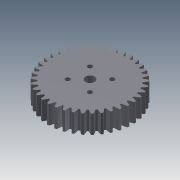
# Autodesk Inventor part: Spur Gear2
Saved by Autodesk Inventor 2015 (Build 190159000, 159)
## iProperties
Created: 2014-08-31
Part Number: Spur Gear2
Material: Steel
Document SubType Name: Modeling
Designer: shohei
Categories: <?xml version="1.0" encoding="UTF-16"?> <MemberInstance><Categories><FamilyTemplate><FamilyTemplateParameter ValueType="xs:double" Id="1" ObjectReferenceKey="da_z" ObjectType="kUserParameterObject"/><FamilyTemplateParameter ValueType="xs:double" Id="2" ObjectReferenceKey="da_b" ObjectType="kUserParameterObject"/><FamilyTemplateParameter ValueType="xs:double" Id="3" ObjectReferenceKey="da_beta" ObjectType="kUserParameterObject"/><FamilyTemplateParameter ValueType="xs:double" Id="4" ObjectReferenceKey="da_da" ObjectType="kUserParameterObject"/><FamilyTemplateParameter ValueType="xs:double" Id="5" ObjectReferenceKey="da_aw" ObjectType="kUserParameterObject"/><FamilyTemplateParameter ValueType="xs:string" Id="6" ObjectReferenceKey="EAIAABAAAACIAQAAAAAAAIAAAAAAAAAA" ObjectType="83910656" SubObjectId="SurfaceGeometry"/></FamilyTemplate><ParamToTemplateMap><ParamToTemplate CategoryParameter="//CategoryParameter[@InternalName='046C89C9-8512-4d59-83FE-43B91F4F132A']" TemplateParameter="1"/><ParamToTemplate CategoryParameter="//CategoryParameter[@InternalName='2552DF32-E462-4b46-AEBF-C6C7768E72AC']" TemplateParameter="2"/><ParamToTemplate CategoryParameter="//CategoryParameter[@InternalName='C9EE641D-15FC-4fae-A226-E94C4372FDD7']" TemplateParameter="3"/><ParamToTemplate><ParamToTemplate CategoryParameter="//CategoryParameter[@InternalName='00B6519A-459B-49c7-AD84-2E56D39A5744']" ConstantValue="0.112596"/></ParamToTemplate><ParamToTemplate><ParamToTemplate CategoryParameter="//CategoryParameter[@InternalName='04B31F0E-C7A6-4894-AA32-9629BEFACF47']" ConstantValue="1.000000"/></ParamToTemplate><ParamToTemplate><ParamToTemplate CategoryParameter="//CategoryParameter[@InternalName='43CBEC2E-7847-49e7-A936-2F7889FCB2D9']" ConstantValue="0.250000"/></ParamToTemplate><ParamToTemplate><ParamToTemplate CategoryParameter="//CategoryParameter[@InternalName='B1EFC894-105D-4ebd-86BF-FA20ED196853']" ConstantValue="0.350000"/></ParamToTemplate><ParamToTemplate><ParamToTemplate CategoryParameter="//CategoryParameter[@InternalName='51175063-3D10-4879-93E8-6246FE8B403D']" ConstantValue="2060000000.000000"/></ParamToTemplate><ParamToTemplate><ParamToTemplate CategoryParameter="//CategoryParameter[@InternalName='A3A52E27-4454-46a9-B0BD-C932399B70AF']" ConstantValue="0.300000"/></ParamToTemplate><ParamToTemplate><ParamToTemplate CategoryParameter="//CategoryParameter[@InternalName='91B76062-C214-41d9-B1B9-14D2AB99603D']" ConstantValue="0.225000"/></ParamToTemplate><ParamToTemplate><ParamToTemplate CategoryParameter="//CategoryParameter[@InternalName='374E806E-8B8A-4dda-A9AA-1039D6500AD2']" ConstantValue="4.444444"/></ParamToTemplate><ParamToTemplate><ParamToTemplate CategoryParameter="//CategoryParameter[@InternalName='2D373A89-B862-43d6-8D0B-0CBF12AB9F6C']" ConstantValue="0.349066"/></ParamToTemplate><ParamToTemplate CategoryParameter="//CategoryParameter[@InternalName='37777632-D6A2-4fac-9D53-DB8ACD95C989']" TemplateParameter="4"/><ParamToTemplate CategoryParameter="//CategoryParameter[@InternalName='FD1017F1-B727-4f7e-9707-0F86F1FF9423']" TemplateParameter="5"/><ParamToTemplate><ParamToTemplate CategoryParameter="//CategoryParameter[@InternalName='9E1B4470-B2D3-4ff1-B813-535BB4CDF51A']" ConstantValue="3520000.000000"/></ParamToTemplate><ParamToTemplate><ParamToTemplate CategoryParameter="//CategoryParameter[@InternalName='F8452263-BFF6-458c-9FB1-07C4B99E95CD']" ConstantValue="11400000.000000"/></ParamToTemplate><ParamToTemplate><ParamToTemplate CategoryParameter="//CategoryParameter[@InternalName='3E3BB259-FD49-497f-8171-6EBC954A3479']" ConstantValue="2.000000"/></ParamToTemplate><ParamToTemplate CategoryParameter="//CategoryParameter[@InternalName='27C3BAF2-7550-4e4b-AE2C-0DB134B7D9B7']" TemplateParameter="6"/></ParamToTemplateMap><Category DisplayName="Gear" InternalName="DC85795E-93AB-48d5-8EEE-5A27447B64BD" Mnemonic="Gear"><CategoryParameter DisplayName="z" InternalName="046C89C9-8512-4d59-83FE-43B91F4F132A" Mnemonic="z"/><CategoryParameter DisplayName="b" InternalName="2552DF32-E462-4b46-AEBF-C6C7768E72AC" Mnemonic="b"/><CategoryParameter DisplayName="||b|" InternalName="C9EE641D-15FC-4fae-A226-E94C4372FDD7" Mnemonic="beta"/><CategoryParameter DisplayName="x" InternalName="00B6519A-459B-49c7-AD84-2E56D39A5744" Mnemonic="x"/><CategoryParameter DisplayName="a*" InternalName="04B31F0E-C7A6-4894-AA32-9629BEFACF47" Mnemonic="a"/><CategoryParameter DisplayName="c*" InternalName="43CBEC2E-7847-49e7-A936-2F7889FCB2D9" Mnemonic="c"/><CategoryParameter DisplayName="r|.f|*" InternalName="B1EFC894-105D-4ebd-86BF-FA20ED196853" Mnemonic="rf"/><CategoryParameter DisplayName="E" InternalName="51175063-3D10-4879-93E8-6246FE8B403D" Mnemonic="E"/><CategoryParameter DisplayName="||m|" InternalName="A3A52E27-4454-46a9-B0BD-C932399B70AF" Mnemonic="mi"/><Category DisplayName="SpurGear" InternalName="26C5A22E-A91E-4dfd-A3B3-23CCAFAE1764" Mnemonic="SpurGear"><CategoryParameter DisplayName="m" InternalName="91B76062-C214-41d9-B1B9-14D2AB99603D" Mnemonic="m"/><CategoryParameter DisplayName="P" InternalName="374E806E-8B8A-4dda-A9AA-1039D6500AD2" Mnemonic="PP"/><CategoryParameter DisplayName="||a|" InternalName="2D373A89-B862-43d6-8D0B-0CBF12AB9F6C" Mnemonic="alpha"/><CategoryParameter DisplayName="d|.a|" InternalName="37777632-D6A2-4fac-9D53-DB8ACD95C989" Mnemonic="da"/><CategoryParameter DisplayName="a|.w|" InternalName="FD1017F1-B727-4f7e-9707-0F86F1FF9423" Mnemonic="aw"/><CategoryParameter DisplayName="||s||.Flim|" InternalName="9E1B4470-B2D3-4ff1-B813-535BB4CDF51A" Mnemonic="sFlim"/><CategoryParameter DisplayName="||s||.Hlim|" InternalName="F8452263-BFF6-458c-9FB1-07C4B99E95CD" Mnemonic="sHlim"/><CategoryParameter DisplayName="type" InternalName="3E3BB259-FD49-497f-8171-6EBC954A3479" Mnemonic="type"/><CategoryParameter DisplayName="PitchDiameter" InternalName="27C3BAF2-7550-4e4b-AE2C-0DB134B7D9B7" Mnemonic="IDS_PITCHDIAM"/></Category></Category></Categories></MemberInstance>
Density: 1 g/cm^3
Appearance: Steel
CustomPartVersion: 1
Author: shohei
Autodesk Inventor part; units mm, degrees
(part 1 of 2)
ref_plane "YZ Plane" through (0, 0, 0) normal (1, 0, 0) x (0, 1, 0)
ref_plane "XZ Plane" through (0, 0, 0) normal (0, 1, 0) x (-1, 0, 0)
ref_plane "XY Plane" through (0, 0, 0) normal (0, 0, 1) x (1, 0, 0)
sketch "Block1" plane through (0, 0, 0) normal (0, 0, 1) x (1, 0, 0)
  arc A0 (1.0814, 45.4571) -> (-1.0814, 45.4571) centre (0, 0) ccw
  arc A1 (2.6745, 40.3222) -> (1.0814, 45.4571) centre (-21.6776, 35.5812) ccw
  arc A2 (3.9987, 40.2125) -> (2.6745, 40.3222) centre (0, 0) ccw
  arc A3 (6.4154, 45.0151) -> (3.9987, 40.2125) centre (27.2384, 31.5279) ccw
  arc A4 (8.5486, 44.6592) -> (6.4154, 45.0151) centre (0, 0) ccw
  arc A5 (9.2749, 39.3321) -> (8.5486, 44.6592) centre (-15.5255, 38.6639) ccw
  arc A6 (10.563, 39.0059) -> (9.2749, 39.3321) centre (0, 0) ccw
  arc A7 (13.7371, 43.3453) -> (10.563, 39.0059) centre (32.0562, 26.6146) ccw
  arc A8 (15.7827, 42.643) -> (13.7371, 43.3453) centre (0, 0) ccw
  arc A9 (15.6222, 37.269) -> (15.7827, 42.643) centre (-8.9499, 40.692) ccw
  arc A10 (16.8391, 36.7353) -> (15.6222, 37.269) centre (0, 0) ccw
  arc A11 (20.6842, 40.493) -> (16.8391, 36.7353) centre (35.9996, 20.9753) ccw
  arc A12 (22.5862, 39.4637) -> (20.6842, 40.493) centre (0, 0) ccw
  arc A13 (21.5435, 34.1894) -> (22.5862, 39.4637) centre (-2.1301, 41.6101) ccw
  arc A14 (22.6558, 33.4627) -> (21.5435, 34.1894) centre (0, 0) ccw
  arc A15 (27.067, 36.5363) -> (22.6558, 33.4627) centre (38.9611, 14.7639) ccw
  arc A16 (28.7737, 35.2079) -> (27.067, 36.5363) centre (0, 0) ccw
  arc A17 (26.877, 30.1772) -> (28.7737, 35.2079) centre (4.7477, 41.3932) ccw
  arc A18 (27.8546, 29.2772) -> (26.877, 30.1772) centre (0, 0) ccw
  arc A19 (32.7115, 31.5829) -> (27.8546, 29.2772) centre (40.8598, 8.1497) ccw
  arc A20 (34.1763, 29.9917) -> (32.7115, 31.5829) centre (0, 0) ccw
  arc A21 (31.4775, 25.3418) -> (34.1763, 29.9917) centre (11.4961, 40.0472) ccw
  arc A22 (32.2936, 24.2932) -> (31.4775, 25.3418) centre (0, 0) ccw
  arc A23 (37.4637, 25.768) -> (32.2936, 24.2932) centre (41.6439, 1.3133) ccw
  arc A24 (38.6466, 23.9574) -> (37.4637, 25.768) centre (0, 0) ccw
  arc A25 (35.2193, 19.8151) -> (38.6466, 23.9574) centre (17.9308, 37.6088) ccw
  arc A26 (35.8517, 18.6465) -> (35.2193, 19.8151) centre (0, 0) ccw
  arc A27 (41.1941, 19.2502) -> (35.8517, 18.6465) centre (41.2921, -5.559) ccw
  arc A28 (42.0628, 17.2696) -> (41.1941, 19.2502) centre (0, 0) ccw
  arc A29 (38.0004, 13.748) -> (42.0628, 17.2696) centre (23.8765, 34.1446) ccw
  arc A30 (38.4318, 12.4912) -> (38.0004, 13.748) centre (0, 0) ccw
  arc A31 (43.8007, 12.2073) -> (38.4318, 12.4912) centre (39.8139, -12.2796) ccw
  arc A32 (44.3316, 10.1108) -> (43.8007, 12.2073) centre (0, 0) ccw
  arc A33 (39.745, 7.3058) -> (44.3316, 10.1108) centre (29.1709, 29.7489) ccw
  arc A34 (39.9637, 5.9952) -> (39.745, 7.3058) centre (0, 0) ccw
  arc A35 (45.2126, 4.8315) -> (39.9637, 5.9952) centre (37.2498, -18.6653) ccw
  arc A36 (45.3912, 2.6762) -> (45.2126, 4.8315) centre (0, 0) ccw
  arc A37 (40.4054, 0.6644) -> (45.3912, 2.6762) centre (33.6695, 24.5418) ccw
  arc A38 (40.4054, -0.6644) -> (40.4054, 0.6644) centre (0, 0) ccw
  arc A39 (45.3912, -2.6762) -> (40.4054, -0.6644) centre (33.6695, -24.5418) ccw
  arc A40 (45.2126, -4.8315) -> (45.3912, -2.6762) centre (0, 0) ccw
  arc A41 (39.9637, -5.9952) -> (45.2126, -4.8315) centre (37.2498, 18.6653) ccw
  arc A42 (39.745, -7.3058) -> (39.9637, -5.9952) centre (0, 0) ccw
  arc A43 (44.3316, -10.1108) -> (39.745, -7.3058) centre (29.1709, -29.7489) ccw
  arc A44 (43.8007, -12.2073) -> (44.3316, -10.1108) centre (0, 0) ccw
  arc A45 (38.4318, -12.4912) -> (43.8007, -12.2073) centre (39.8139, 12.2796) ccw
  arc A46 (38.0004, -13.748) -> (38.4318, -12.4912) centre (0, 0) ccw
  arc A47 (42.0628, -17.2696) -> (38.0004, -13.748) centre (23.8765, -34.1446) ccw
  arc A48 (41.1941, -19.2502) -> (42.0628, -17.2696) centre (0, 0) ccw
  arc A49 (35.8517, -18.6465) -> (41.1941, -19.2502) centre (41.2921, 5.559) ccw
  arc A50 (35.2193, -19.8151) -> (35.8517, -18.6465) centre (0, 0) ccw
  arc A51 (38.6466, -23.9574) -> (35.2193, -19.8151) centre (17.9308, -37.6088) ccw
  arc A52 (37.4637, -25.768) -> (38.6466, -23.9574) centre (0, 0) ccw
  arc A53 (32.2936, -24.2932) -> (37.4637, -25.768) centre (41.6439, -1.3133) ccw
  arc A54 (31.4775, -25.3418) -> (32.2936, -24.2932) centre (0, 0) ccw
  arc A55 (34.1763, -29.9917) -> (31.4775, -25.3418) centre (11.4961, -40.0472) ccw
  arc A56 (32.7115, -31.5829) -> (34.1763, -29.9917) centre (0, 0) ccw
  arc A57 (27.8546, -29.2772) -> (32.7115, -31.5829) centre (40.8598, -8.1497) ccw
  arc A58 (26.877, -30.1772) -> (27.8546, -29.2772) centre (0, 0) ccw
  arc A59 (28.7737, -35.2079) -> (26.877, -30.1772) centre (4.7477, -41.3932) ccw
  arc A60 (27.067, -36.5363) -> (28.7737, -35.2079) centre (0, 0) ccw
  arc A61 (22.6558, -33.4627) -> (27.067, -36.5363) centre (38.9611, -14.7639) ccw
  arc A62 (21.5435, -34.1894) -> (22.6558, -33.4627) centre (0, 0) ccw
  arc A63 (22.5862, -39.4637) -> (21.5435, -34.1894) centre (-2.1301, -41.6101) ccw
  arc A64 (20.6842, -40.493) -> (22.5862, -39.4637) centre (0, 0) ccw
  arc A65 (16.8391, -36.7353) -> (20.6842, -40.493) centre (35.9996, -20.9753) ccw
  arc A66 (15.6222, -37.269) -> (16.8391, -36.7353) centre (0, 0) ccw
  arc A67 (15.7827, -42.643) -> (15.6222, -37.269) centre (-8.9499, -40.692) ccw
  arc A68 (13.7371, -43.3453) -> (15.7827, -42.643) centre (0, 0) ccw
  arc A69 (10.563, -39.0059) -> (13.7371, -43.3453) centre (32.0562, -26.6146) ccw
  arc A70 (9.2749, -39.3321) -> (10.563, -39.0059) centre (0, 0) ccw
  arc A71 (8.5486, -44.6592) -> (9.2749, -39.3321) centre (-15.5255, -38.6639) ccw
  arc A72 (6.4154, -45.0151) -> (8.5486, -44.6592) centre (0, 0) ccw
  arc A73 (3.9987, -40.2125) -> (6.4154, -45.0151) centre (27.2384, -31.5279) ccw
  arc A74 (2.6745, -40.3222) -> (3.9987, -40.2125) centre (0, 0) ccw
  arc A75 (1.0814, -45.4571) -> (2.6745, -40.3222) centre (-21.6776, -35.5812) ccw
  arc A76 (-1.0814, -45.4571) -> (1.0814, -45.4571) centre (0, 0) ccw
  arc A77 (-2.6745, -40.3222) -> (-1.0814, -45.4571) centre (21.6776, -35.5812) ccw
  arc A78 (-3.9987, -40.2125) -> (-2.6745, -40.3222) centre (0, 0) ccw
  arc A79 (-6.4154, -45.0151) -> (-3.9987, -40.2125) centre (-27.2384, -31.5279) ccw
  arc A80 (-8.5486, -44.6592) -> (-6.4154, -45.0151) centre (0, 0) ccw
  arc A81 (-9.2749, -39.3321) -> (-8.5486, -44.6592) centre (15.5255, -38.6639) ccw
  arc A82 (-10.563, -39.0059) -> (-9.2749, -39.3321) centre (0, 0) ccw
  arc A83 (-13.7371, -43.3453) -> (-10.563, -39.0059) centre (-32.0562, -26.6146) ccw
  arc A84 (-15.7827, -42.643) -> (-13.7371, -43.3453) centre (0, 0) ccw
  arc A85 (-15.6222, -37.269) -> (-15.7827, -42.643) centre (8.9499, -40.692) ccw
  arc A86 (-16.8391, -36.7353) -> (-15.6222, -37.269) centre (0, 0) ccw
  arc A87 (-20.6842, -40.493) -> (-16.8391, -36.7353) centre (-35.9996, -20.9753) ccw
  arc A88 (-22.5862, -39.4637) -> (-20.6842, -40.493) centre (0, 0) ccw
  arc A89 (-21.5435, -34.1894) -> (-22.5862, -39.4637) centre (2.1301, -41.6101) ccw
  arc A90 (-22.6558, -33.4627) -> (-21.5435, -34.1894) centre (0, 0) ccw
  arc A91 (-27.067, -36.5363) -> (-22.6558, -33.4627) centre (-38.9611, -14.7639) ccw
  arc A92 (-28.7737, -35.2079) -> (-27.067, -36.5363) centre (0, 0) ccw
  arc A93 (-26.877, -30.1772) -> (-28.7737, -35.2079) centre (-4.7477, -41.3932) ccw
  arc A94 (-27.8546, -29.2772) -> (-26.877, -30.1772) centre (0, 0) ccw
  arc A95 (-32.7115, -31.5829) -> (-27.8546, -29.2772) centre (-40.8598, -8.1497) ccw
  arc A96 (-34.1763, -29.9917) -> (-32.7115, -31.5829) centre (0, 0) ccw
  arc A97 (-31.4775, -25.3418) -> (-34.1763, -29.9917) centre (-11.4961, -40.0472) ccw
  arc A98 (-32.2936, -24.2932) -> (-31.4775, -25.3418) centre (0, 0) ccw
  arc A99 (-37.4637, -25.768) -> (-32.2936, -24.2932) centre (-41.6439, -1.3133) ccw
  arc A100 (-38.6466, -23.9574) -> (-37.4637, -25.768) centre (0, 0) ccw
  arc A101 (-35.2193, -19.8151) -> (-38.6466, -23.9574) centre (-17.9308, -37.6088) ccw
  arc A102 (-35.8517, -18.6465) -> (-35.2193, -19.8151) centre (0, 0) ccw
  arc A103 (-41.1941, -19.2502) -> (-35.8517, -18.6465) centre (-41.2921, 5.559) ccw
  arc A104 (-42.0628, -17.2696) -> (-41.1941, -19.2502) centre (0, 0) ccw
  arc A105 (-38.0004, -13.748) -> (-42.0628, -17.2696) centre (-23.8765, -34.1446) ccw
  arc A106 (-38.4318, -12.4912) -> (-38.0004, -13.748) centre (0, 0) ccw
  arc A107 (-43.8007, -12.2073) -> (-38.4318, -12.4912) centre (-39.8139, 12.2796) ccw
  arc A108 (-44.3316, -10.1108) -> (-43.8007, -12.2073) centre (0, 0) ccw
  arc A109 (-39.745, -7.3058) -> (-44.3316, -10.1108) centre (-29.1709, -29.7489) ccw
  arc A110 (-39.9637, -5.9952) -> (-39.745, -7.3058) centre (0, 0) ccw
  arc A111 (-45.2126, -4.8315) -> (-39.9637, -5.9952) centre (-37.2498, 18.6653) ccw
  arc A112 (-45.3912, -2.6762) -> (-45.2126, -4.8315) centre (0, 0) ccw
  arc A113 (-40.4054, -0.6644) -> (-45.3912, -2.6762) centre (-33.6695, -24.5418) ccw
  arc A114 (-40.4054, 0.6644) -> (-40.4054, -0.6644) centre (0, 0) ccw
  arc A115 (-45.3912, 2.6762) -> (-40.4054, 0.6644) centre (-33.6695, 24.5418) ccw
  arc A116 (-45.2126, 4.8315) -> (-45.3912, 2.6762) centre (0, 0) ccw
  arc A117 (-39.9637, 5.9952) -> (-45.2126, 4.8315) centre (-37.2498, -18.6653) ccw
  arc A118 (-39.745, 7.3058) -> (-39.9637, 5.9952) centre (0, 0) ccw
  arc A119 (-44.3316, 10.1108) -> (-39.745, 7.3058) centre (-29.1709, 29.7489) ccw
  arc A120 (-43.8007, 12.2073) -> (-44.3316, 10.1108) centre (0, 0) ccw
  arc A121 (-38.4318, 12.4912) -> (-43.8007, 12.2073) centre (-39.8139, -12.2796) ccw
  arc A122 (-38.0004, 13.748) -> (-38.4318, 12.4912) centre (0, 0) ccw
  arc A123 (-42.0628, 17.2696) -> (-38.0004, 13.748) centre (-23.8765, 34.1446) ccw
  arc A124 (-41.1941, 19.2502) -> (-42.0628, 17.2696) centre (0, 0) ccw
  arc A125 (-35.8517, 18.6465) -> (-41.1941, 19.2502) centre (-41.2921, -5.559) ccw
  arc A126 (-35.2193, 19.8151) -> (-35.8517, 18.6465) centre (0, 0) ccw
  arc A127 (-38.6466, 23.9574) -> (-35.2193, 19.8151) centre (-17.9308, 37.6088) ccw
  arc A128 (-37.4637, 25.768) -> (-38.6466, 23.9574) centre (0, 0) ccw
  arc A129 (-32.2936, 24.2932) -> (-37.4637, 25.768) centre (-41.6439, 1.3133) ccw
  arc A130 (-31.4775, 25.3418) -> (-32.2936, 24.2932) centre (0, 0) ccw
  arc A131 (-34.1763, 29.9917) -> (-31.4775, 25.3418) centre (-11.4961, 40.0472) ccw
  arc A132 (-32.7115, 31.5829) -> (-34.1763, 29.9917) centre (0, 0) ccw
  arc A133 (-27.8546, 29.2772) -> (-32.7115, 31.5829) centre (-40.8598, 8.1497) ccw
  arc A134 (-26.877, 30.1772) -> (-27.8546, 29.2772) centre (0, 0) ccw
  arc A135 (-28.7737, 35.2079) -> (-26.877, 30.1772) centre (-4.7477, 41.3932) ccw
  arc A136 (-27.067, 36.5363) -> (-28.7737, 35.2079) centre (0, 0) ccw
  arc A137 (-22.6558, 33.4627) -> (-27.067, 36.5363) centre (-38.9611, 14.7639) ccw
  arc A138 (-21.5435, 34.1894) -> (-22.6558, 33.4627) centre (0, 0) ccw
  arc A139 (-22.5862, 39.4637) -> (-21.5435, 34.1894) centre (2.1301, 41.6101) ccw
  arc A140 (-20.6842, 40.493) -> (-22.5862, 39.4637) centre (0, 0) ccw
  arc A141 (-16.8391, 36.7353) -> (-20.6842, 40.493) centre (-35.9996, 20.9753) ccw
  arc A142 (-15.6222, 37.269) -> (-16.8391, 36.7353) centre (0, 0) ccw
  arc A143 (-15.7827, 42.643) -> (-15.6222, 37.269) centre (8.9499, 40.692) ccw
  arc A144 (-13.7371, 43.3453) -> (-15.7827, 42.643) centre (0, 0) ccw
  arc A145 (-10.563, 39.0059) -> (-13.7371, 43.3453) centre (-32.0562, 26.6146) ccw
  arc A146 (-9.2749, 39.3321) -> (-10.563, 39.0059) centre (0, 0) ccw
  arc A147 (-8.5486, 44.6592) -> (-9.2749, 39.3321) centre (15.5255, 38.6639) ccw
  arc A148 (-6.4154, 45.0151) -> (-8.5486, 44.6592) centre (0, 0) ccw
  arc A149 (-3.9987, 40.2125) -> (-6.4154, 45.0151) centre (-27.2384, 31.5279) ccw
  arc A150 (-2.6745, 40.3222) -> (-3.9987, 40.2125) centre (0, 0) ccw
  arc A151 (-1.0814, 45.4571) -> (-2.6745, 40.3222) centre (21.6776, 35.5812) ccw
  circle A152 centre (-12, 12) radius 2.72
  circle A153 centre (0, 0) radius 5.22
  circle A154 centre (-12, -12) radius 2.72
  circle A155 centre (12, 12) radius 2.72
  circle A156 centre (12, -12) radius 2.72
  point P0 (0, 0)
sketch "Sketch1" plane through (0, 0, 0) normal (0, 0, 1) x (1, 0, 0)
  circle A0 centre (0, 0) radius 45.25
  line L0 (-63.35, 0) -> (63.35, 0) projected
  line L1 (0, -63.35) -> (0, 63.35) projected
  circle A1 centre (-15, 15) radius 2.5
  dimension "d0" = 90.5
  dimension "d52" = 5
  dimension "d53" = 15
  dimension "d54" = 15
  constraints: 2 centre point
  measures "d0" diameter of A0
  measures "d52" diameter of A1
  measures "d53" distance from line of L1 A1.centre
  measures "d54" distance from line of L0 A1.centre
extrude "Extrusion1" add sketch "Sketch1" along normal blind 20 contours L0 L1 A0 | A0 L1 L0 | L1 L0 A0 | A0 L0 L1 | A1
ref_plane "Work Plane2" through (0, 0, 10) normal (0, 0, 1) x (1, 0, 0)
sketch "Sketch2" plane through (0, 0, 0) normal (0, 0, -1) x (-1, 0, 0)
  circle A0 centre (0, 0) radius 45.25 projected
  circle A1 centre (0, 0) radius 42.9032
  dimension "d3" = 85.8064
  constraints: 1 centre point, 1 coincident
  measures "d3" diameter of A1
surface extrude "Pitch Diameter" sketch "Sketch2" against normal through all shown no curves A1
ref_plane "Work Plane8" through (0, 0, 0) normal (0.9965845, 0.0825793, 0) x (0, 0, 1)
ref_plane "Work Plane9" through (0, 0, 0) normal (1, 0, 0) x (0, 1, 0)
spur gear teeth "Spur Gear" teeth 38 pitch diameter 85.5 tip diameter 90.5 root diameter 80.3817 face width 20 start plane through (0, 0, 0) normal (0, 0, -1) x (-1, 0, 0)
sketch "Sketch3" plane through (0, 0, 0) normal (0, 0, -1) x (-1, 0, 0)
  circle A0 centre (0, 0) radius 5
  line L0 (63.2283, 0) -> (-63.2283, 0) projected
  line L1 (0, -63.35) -> (0, 63.35) projected
  circle A1 centre (12, 12) radius 2.5
  circle A2 centre (12, -12) radius 2.5
  circle A3 centre (-12, 12) radius 2.5
  circle A4 centre (-12, -12) radius 2.5
  dimension "d51" = 10
  dimension "d55" = 5
  dimension "d56" = 12
  dimension "d57" = 12
  constraints: 5 centre point, 3 symmetric about line, 1 coincident, 3 other
  measures "d51" diameter of A0
  measures "d55" diameter of A1
  measures "d56" distance from line of L0 A1.centre
  measures "d57" distance from line of L1 A1.centre
extrude "Extrusion3" cut sketch "Sketch3" against normal through all
sketch "Sketch4" plane through (0, 0, 20) normal (0, 0, 1) x (1, 0, 0)
  circle A0 centre (12, -12) radius 2.5 projected
  circle A1 centre (-12, -12) radius 2.5 projected
  circle A2 centre (-12, 12) radius 2.5 projected
  circle A3 centre (12, 12) radius 2.5 projected
  circle A4 centre (0, 0) radius 5 projected
  arc A5 (-8.3687, 44.4694) -> (-9.059, 39.1566) centre (15.5255, 38.6639) ccw projected
  arc A6 (-9.059, 39.1566) -> (-10.6694, 38.7488) centre (0, 0) ccw projected
  arc A7 (-10.6694, 38.7488) -> (-13.805, 43.0927) centre (-32.0562, 26.6146) ccw projected
  arc A8 (-13.805, 43.0927) -> (-15.574, 42.4854) centre (0, 0) ccw projected
  arc A9 (-15.574, 42.4854) -> (-15.3804, 37.1315) centre (8.9499, 40.692) ccw projected
  arc A10 (-15.3804, 37.1315) -> (-16.9017, 36.4642) centre (0, 0) ccw projected
  arc A11 (-16.9017, 36.4642) -> (-20.7096, 40.2328) centre (-35.9996, 20.9753) ccw projected
  arc A12 (-20.7096, 40.2328) -> (-22.3545, 39.3426) centre (0, 0) ccw projected
  arc A13 (-22.3545, 39.3426) -> (-21.2822, 34.0935) centre (2.1301, 41.6101) ccw projected
  arc A14 (-21.2822, 34.0935) -> (-22.673, 33.1849) centre (0, 0) ccw projected
  arc A15 (-22.673, 33.1849) -> (-27.0492, 36.2754) centre (-38.9611, 14.7639) ccw projected
  arc A16 (-27.0492, 36.2754) -> (-28.5252, 35.1266) centre (0, 0) ccw projected
  arc A17 (-28.5252, 35.1266) -> (-26.6036, 30.1256) centre (-4.7477, 41.3932) ccw projected
  arc A18 (-26.6036, 30.1256) -> (-27.8258, 29.0005) centre (0, 0) ccw projected
  arc A19 (-27.8258, 29.0005) -> (-32.651, 31.3285) centre (-40.8598, 8.1497) ccw projected
  arc A20 (-32.651, 31.3285) -> (-33.9178, 29.9524) centre (0, 0) ccw projected
  arc A21 (-33.9178, 29.9524) -> (-31.1993, 25.3359) centre (-11.4961, 40.0472) ccw projected
  arc A22 (-31.1993, 25.3359) -> (-32.2196, 24.025) centre (0, 0) ccw projected
  arc A23 (-32.2196, 24.025) -> (-37.3622, 25.527) centre (-41.6439, 1.3133) ccw projected
  arc A24 (-37.3622, 25.527) -> (-38.3852, 23.9612) centre (0, 0) ccw projected
  arc A25 (-38.3852, 23.9612) -> (-34.9439, 19.8551) centre (-17.9308, 37.6088) ccw projected
  arc A26 (-34.9439, 19.8551) -> (-35.7346, 18.3941) centre (0, 0) ccw projected
  arc A27 (-35.7346, 18.3941) -> (-41.0542, 19.0292) centre (-41.2921, -5.559) ccw projected
  arc A28 (-41.0542, 19.0292) -> (-41.8055, 17.3164) centre (0, 0) ccw projected
  arc A29 (-41.8055, 17.3164) -> (-37.7354, 13.8328) centre (-23.8765, 34.1446) ccw projected
  arc A30 (-37.7354, 13.8328) -> (-38.2748, 12.2615) centre (0, 0) ccw projected
  arc A31 (-38.2748, 12.2615) -> (-43.6264, 12.0124) centre (-39.8139, -12.2796) ccw projected
  arc A32 (-43.6264, 12.0124) -> (-44.0856, 10.1993) centre (0, 0) ccw projected
  arc A33 (-44.0856, 10.1993) -> (-39.4975, 7.4331) centre (-29.1709, 29.7489) ccw projected
  arc A34 (-39.4975, 7.4331) -> (-39.7709, 5.7945) centre (0, 0) ccw projected
  arc A35 (-39.7709, 5.7945) -> (-45.0086, 4.6679) centre (-37.2498, -18.6653) ccw projected
  arc A36 (-45.0086, 4.6679) -> (-45.163, 2.8039) centre (0, 0) ccw projected
  arc A37 (-45.163, 2.8039) -> (-40.1823, 0.8306) centre (-33.6695, 24.5418) ccw projected
  arc A38 (-40.1823, 0.8306) -> (-40.1823, -0.8306) centre (0, 0) ccw projected
  arc A39 (-40.1823, -0.8306) -> (-45.163, -2.8039) centre (-33.6695, -24.5418) ccw projected
  arc A40 (-45.163, -2.8039) -> (-45.0086, -4.6679) centre (0, 0) ccw projected
  arc A41 (-45.0086, -4.6679) -> (-39.7709, -5.7945) centre (-37.2498, 18.6653) ccw projected
  arc A42 (-39.7709, -5.7945) -> (-39.4975, -7.4331) centre (0, 0) ccw projected
  arc A43 (-39.4975, -7.4331) -> (-44.0856, -10.1993) centre (-29.1709, -29.7489) ccw projected
  arc A44 (-44.0856, -10.1993) -> (-43.6264, -12.0124) centre (0, 0) ccw projected
  arc A45 (-43.6264, -12.0124) -> (-38.2748, -12.2615) centre (-39.8139, 12.2796) ccw projected
  arc A46 (-38.2748, -12.2615) -> (-37.7354, -13.8328) centre (0, 0) ccw projected
  arc A47 (-37.7354, -13.8328) -> (-41.8055, -17.3164) centre (-23.8765, -34.1446) ccw projected
  arc A48 (-41.8055, -17.3164) -> (-41.0542, -19.0292) centre (0, 0) ccw projected
  arc A49 (-41.0542, -19.0292) -> (-35.7346, -18.3941) centre (-41.2921, 5.559) ccw projected
  arc A50 (-35.7346, -18.3941) -> (-34.9439, -19.8551) centre (0, 0) ccw projected
  arc A51 (-34.9439, -19.8551) -> (-38.3852, -23.9612) centre (-17.9308, -37.6088) ccw projected
  arc A52 (-38.3852, -23.9612) -> (-37.3622, -25.527) centre (0, 0) ccw projected
  arc A53 (-37.3622, -25.527) -> (-32.2196, -24.025) centre (-41.6439, -1.3133) ccw projected
  arc A54 (-32.2196, -24.025) -> (-31.1993, -25.3359) centre (0, 0) ccw projected
  arc A55 (-31.1993, -25.3359) -> (-33.9178, -29.9524) centre (-11.4961, -40.0472) ccw projected
  arc A56 (-33.9178, -29.9524) -> (-32.651, -31.3285) centre (0, 0) ccw projected
  arc A57 (-32.651, -31.3285) -> (-27.8258, -29.0005) centre (-40.8598, -8.1497) ccw projected
  arc A58 (-27.8258, -29.0005) -> (-26.6036, -30.1256) centre (0, 0) ccw projected
  arc A59 (-26.6036, -30.1256) -> (-28.5252, -35.1266) centre (-4.7477, -41.3932) ccw projected
  arc A60 (-28.5252, -35.1266) -> (-27.0492, -36.2754) centre (0, 0) ccw projected
  arc A61 (-27.0492, -36.2754) -> (-22.673, -33.1849) centre (-38.9611, -14.7639) ccw projected
  arc A62 (-22.673, -33.1849) -> (-21.2822, -34.0935) centre (0, 0) ccw projected
  arc A63 (-21.2822, -34.0935) -> (-22.3545, -39.3426) centre (2.1301, -41.6101) ccw projected
  arc A64 (-22.3545, -39.3426) -> (-20.7096, -40.2328) centre (0, 0) ccw projected
  arc A65 (-20.7096, -40.2328) -> (-16.9017, -36.4642) centre (-35.9996, -20.9753) ccw projected
  arc A66 (-16.9017, -36.4642) -> (-15.3804, -37.1315) centre (0, 0) ccw projected
  arc A67 (-15.3804, -37.1315) -> (-15.574, -42.4854) centre (8.9499, -40.692) ccw projected
  arc A68 (-15.574, -42.4854) -> (-13.805, -43.0927) centre (0, 0) ccw projected
  arc A69 (-13.805, -43.0927) -> (-10.6694, -38.7488) centre (-32.0562, -26.6146) ccw projected
  arc A70 (-10.6694, -38.7488) -> (-9.059, -39.1566) centre (0, 0) ccw projected
  arc A71 (-9.059, -39.1566) -> (-8.3687, -44.4694) centre (15.5255, -38.6639) ccw projected
  arc A72 (-8.3687, -44.4694) -> (-6.5239, -44.7772) centre (0, 0) ccw projected
  arc A73 (-6.5239, -44.7772) -> (-4.146, -39.9764) centre (-27.2384, -31.5279) ccw projected
  arc A74 (-4.146, -39.9764) -> (-2.4904, -40.1136) centre (0, 0) ccw projected
  arc A75 (-2.4904, -40.1136) -> (-0.9352, -45.2403) centre (21.6776, -35.5812) ccw projected
  arc A76 (-0.9352, -45.2403) -> (0.9352, -45.2403) centre (0, 0) ccw projected
  arc A77 (0.9352, -45.2403) -> (2.4904, -40.1136) centre (-21.6776, -35.5812) ccw projected
  arc A78 (2.4904, -40.1136) -> (4.146, -39.9764) centre (0, 0) ccw projected
  arc A79 (4.146, -39.9764) -> (6.5239, -44.7772) centre (27.2384, -31.5279) ccw projected
  arc A80 (6.5239, -44.7772) -> (8.3687, -44.4694) centre (0, 0) ccw projected
  arc A81 (8.3687, -44.4694) -> (9.059, -39.1566) centre (-15.5255, -38.6639) ccw projected
  arc A82 (9.059, -39.1566) -> (10.6694, -38.7488) centre (0, 0) ccw projected
  arc A83 (10.6694, -38.7488) -> (13.805, -43.0927) centre (32.0562, -26.6146) ccw projected
  arc A84 (13.805, -43.0927) -> (15.574, -42.4854) centre (0, 0) ccw projected
  arc A85 (15.574, -42.4854) -> (15.3804, -37.1315) centre (-8.9499, -40.692) ccw projected
  arc A86 (15.3804, -37.1315) -> (16.9017, -36.4642) centre (0, 0) ccw projected
  arc A87 (16.9017, -36.4642) -> (20.7096, -40.2328) centre (35.9996, -20.9753) ccw projected
  arc A88 (20.7096, -40.2328) -> (22.3545, -39.3426) centre (0, 0) ccw projected
  arc A89 (22.3545, -39.3426) -> (21.2822, -34.0935) centre (-2.1301, -41.6101) ccw projected
  arc A90 (21.2822, -34.0935) -> (22.673, -33.1849) centre (0, 0) ccw projected
  arc A91 (22.673, -33.1849) -> (27.0492, -36.2754) centre (38.9611, -14.7639) ccw projected
  arc A92 (27.0492, -36.2754) -> (28.5252, -35.1266) centre (0, 0) ccw projected
  arc A93 (28.5252, -35.1266) -> (26.6036, -30.1256) centre (4.7477, -41.3932) ccw projected
  arc A94 (26.6036, -30.1256) -> (27.8258, -29.0005) centre (0, 0) ccw projected
  arc A95 (27.8258, -29.0005) -> (32.651, -31.3285) centre (40.8598, -8.1497) ccw projected
  arc A96 (32.651, -31.3285) -> (33.9178, -29.9524) centre (0, 0) ccw projected
  arc A97 (33.9178, -29.9524) -> (31.1993, -25.3359) centre (11.4961, -40.0472) ccw projected
  arc A98 (31.1993, -25.3359) -> (32.2196, -24.025) centre (0, 0) ccw projected
  arc A99 (32.2196, -24.025) -> (37.3622, -25.527) centre (41.6439, -1.3133) ccw projected
  arc A100 (37.3622, -25.527) -> (38.3852, -23.9612) centre (0, 0) ccw projected
  arc A101 (38.3852, -23.9612) -> (34.9439, -19.8551) centre (17.9308, -37.6088) ccw projected
  arc A102 (34.9439, -19.8551) -> (35.7346, -18.3941) centre (0, 0) ccw projected
  arc A103 (35.7346, -18.3941) -> (41.0542, -19.0292) centre (41.2921, 5.559) ccw projected
  arc A104 (41.0542, -19.0292) -> (41.8055, -17.3164) centre (0, 0) ccw projected
  arc A105 (41.8055, -17.3164) -> (37.7354, -13.8328) centre (23.8765, -34.1446) ccw projected
  arc A106 (37.7354, -13.8328) -> (38.2748, -12.2615) centre (0, 0) ccw projected
  arc A107 (38.2748, -12.2615) -> (43.6264, -12.0124) centre (39.8139, 12.2796) ccw projected
  arc A108 (43.6264, -12.0124) -> (44.0856, -10.1993) centre (0, 0) ccw projected
  arc A109 (44.0856, -10.1993) -> (39.4975, -7.4331) centre (29.1709, -29.7489) ccw projected
  arc A110 (39.4975, -7.4331) -> (39.7709, -5.7945) centre (0, 0) ccw projected
  arc A111 (39.7709, -5.7945) -> (45.0086, -4.6679) centre (37.2498, 18.6653) ccw projected
  arc A112 (45.0086, -4.6679) -> (45.163, -2.8039) centre (0, 0) ccw projected
  arc A113 (45.163, -2.8039) -> (40.1823, -0.8306) centre (33.6695, -24.5418) ccw projected
  arc A114 (40.1823, -0.8306) -> (40.1823, 0.8306) centre (0, 0) ccw projected
  arc A115 (40.1823, 0.8306) -> (45.163, 2.8039) centre (33.6695, 24.5418) ccw projected
  arc A116 (45.163, 2.8039) -> (45.0086, 4.6679) centre (0, 0) ccw projected
  arc A117 (45.0086, 4.6679) -> (39.7709, 5.7945) centre (37.2498, -18.6653) ccw projected
  arc A118 (39.7709, 5.7945) -> (39.4975, 7.4331) centre (0, 0) ccw projected
  arc A119 (39.4975, 7.4331) -> (44.0856, 10.1993) centre (29.1709, 29.7489) ccw projected
  arc A120 (44.0856, 10.1993) -> (43.6264, 12.0124) centre (0, 0) ccw projected
  arc A121 (43.6264, 12.0124) -> (38.2748, 12.2615) centre (39.8139, -12.2796) ccw projected
  arc A122 (38.2748, 12.2615) -> (37.7354, 13.8328) centre (0, 0) ccw projected
  arc A123 (37.7354, 13.8328) -> (41.8055, 17.3164) centre (23.8765, 34.1446) ccw projected
  arc A124 (41.8055, 17.3164) -> (41.0542, 19.0292) centre (0, 0) ccw projected
  arc A125 (41.0542, 19.0292) -> (35.7346, 18.3941) centre (41.2921, -5.559) ccw projected
  arc A126 (35.7346, 18.3941) -> (34.9439, 19.8551) centre (0, 0) ccw projected
  arc A127 (34.9439, 19.8551) -> (38.3852, 23.9612) centre (17.9308, 37.6088) ccw projected
  arc A128 (38.3852, 23.9612) -> (37.3622, 25.527) centre (0, 0) ccw projected
  arc A129 (37.3622, 25.527) -> (32.2196, 24.025) centre (41.6439, 1.3133) ccw projected
  arc A130 (32.2196, 24.025) -> (31.1993, 25.3359) centre (0, 0) ccw projected
  arc A131 (31.1993, 25.3359) -> (33.9178, 29.9524) centre (11.4961, 40.0472) ccw projected
  arc A132 (33.9178, 29.9524) -> (32.651, 31.3285) centre (0, 0) ccw projected
  arc A133 (32.651, 31.3285) -> (27.8258, 29.0005) centre (40.8598, 8.1497) ccw projected
  arc A134 (27.8258, 29.0005) -> (26.6036, 30.1256) centre (0, 0) ccw projected
  arc A135 (26.6036, 30.1256) -> (28.5252, 35.1266) centre (4.7477, 41.3932) ccw projected
  arc A136 (28.5252, 35.1266) -> (27.0492, 36.2754) centre (0, 0) ccw projected
  arc A137 (27.0492, 36.2754) -> (22.673, 33.1849) centre (38.9611, 14.7639) ccw projected
  arc A138 (22.673, 33.1849) -> (21.2822, 34.0935) centre (0, 0) ccw projected
  arc A139 (21.2822, 34.0935) -> (22.3545, 39.3426) centre (-2.1301, 41.6101) ccw projected
  arc A140 (22.3545, 39.3426) -> (20.7096, 40.2328) centre (0, 0) ccw projected
  arc A141 (20.7096, 40.2328) -> (16.9017, 36.4642) centre (35.9996, 20.9753) ccw projected
  arc A142 (16.9017, 36.4642) -> (15.3804, 37.1315) centre (0, 0) ccw projected
  arc A143 (15.3804, 37.1315) -> (15.574, 42.4854) centre (-8.9499, 40.692) ccw projected
  arc A144 (15.574, 42.4854) -> (13.805, 43.0927) centre (0, 0) ccw projected
  arc A145 (13.805, 43.0927) -> (10.6694, 38.7488) centre (32.0562, 26.6146) ccw projected
  arc A146 (10.6694, 38.7488) -> (9.059, 39.1566) centre (0, 0) ccw projected
  arc A147 (9.059, 39.1566) -> (8.3687, 44.4694) centre (-15.5255, 38.6639) ccw projected
  arc A148 (8.3687, 44.4694) -> (6.5239, 44.7772) centre (0, 0) ccw projected
  arc A149 (6.5239, 44.7772) -> (4.146, 39.9764) centre (27.2384, 31.5279) ccw projected
  arc A150 (4.146, 39.9764) -> (2.4904, 40.1136) centre (0, 0) ccw projected
  arc A151 (2.4904, 40.1136) -> (0.9352, 45.2403) centre (-21.6776, 35.5812) ccw projected
  arc A152 (0.9352, 45.2403) -> (-0.9352, 45.2403) centre (0, 0) ccw projected
  arc A153 (-0.9352, 45.2403) -> (-2.4904, 40.1136) centre (21.6776, 35.5812) ccw projected
  arc A154 (-2.4904, 40.1136) -> (-4.146, 39.9764) centre (0, 0) ccw projected
  arc A155 (-4.146, 39.9764) -> (-6.5239, 44.7772) centre (-27.2384, 31.5279) ccw projected
  arc A156 (-6.5239, 44.7772) -> (-8.3687, 44.4694) centre (0, 0) ccw projected
  arc A157 (1.0814, 45.4571) -> (-1.0814, 45.4571) centre (0, 0) ccw
  arc A158 (2.6745, 40.3222) -> (1.0814, 45.4571) centre (-21.6776, 35.5812) ccw
  arc A159 (3.9987, 40.2125) -> (2.6745, 40.3222) centre (0, 0) ccw
  arc A160 (6.4154, 45.0151) -> (3.9987, 40.2125) centre (27.2384, 31.5279) ccw
  arc A161 (8.5486, 44.6592) -> (6.4154, 45.0151) centre (0, 0) ccw
  arc A162 (9.2749, 39.3321) -> (8.5486, 44.6592) centre (-15.5255, 38.6639) ccw
  arc A163 (10.563, 39.0059) -> (9.2749, 39.3321) centre (0, 0) ccw
  arc A164 (13.7371, 43.3453) -> (10.563, 39.0059) centre (32.0562, 26.6146) ccw
  arc A165 (15.7827, 42.643) -> (13.7371, 43.3453) centre (0, 0) ccw
  arc A166 (15.6222, 37.269) -> (15.7827, 42.643) centre (-8.9499, 40.692) ccw
  arc A167 (16.8391, 36.7353) -> (15.6222, 37.269) centre (0, 0) ccw
  arc A168 (20.6842, 40.493) -> (16.8391, 36.7353) centre (35.9996, 20.9753) ccw
  arc A169 (22.5862, 39.4637) -> (20.6842, 40.493) centre (0, 0) ccw
  arc A170 (21.5435, 34.1894) -> (22.5862, 39.4637) centre (-2.1301, 41.6101) ccw
  arc A171 (22.6558, 33.4627) -> (21.5435, 34.1894) centre (0, 0) ccw
  arc A172 (27.067, 36.5363) -> (22.6558, 33.4627) centre (38.9611, 14.7639) ccw
  arc A173 (28.7737, 35.2079) -> (27.067, 36.5363) centre (0, 0) ccw
  arc A174 (26.877, 30.1772) -> (28.7737, 35.2079) centre (4.7477, 41.3932) ccw
  arc A175 (27.8546, 29.2772) -> (26.877, 30.1772) centre (0, 0) ccw
  arc A176 (32.7115, 31.5829) -> (27.8546, 29.2772) centre (40.8598, 8.1497) ccw
  arc A177 (34.1763, 29.9917) -> (32.7115, 31.5829) centre (0, 0) ccw
  arc A178 (31.4775, 25.3418) -> (34.1763, 29.9917) centre (11.4961, 40.0472) ccw
  arc A179 (32.2936, 24.2932) -> (31.4775, 25.3418) centre (0, 0) ccw
  arc A180 (37.4637, 25.768) -> (32.2936, 24.2932) centre (41.6439, 1.3133) ccw
  arc A181 (38.6466, 23.9574) -> (37.4637, 25.768) centre (0, 0) ccw
  arc A182 (35.2193, 19.8151) -> (38.6466, 23.9574) centre (17.9308, 37.6088) ccw
  arc A183 (35.8517, 18.6465) -> (35.2193, 19.8151) centre (0, 0) ccw
  arc A184 (41.1941, 19.2502) -> (35.8517, 18.6465) centre (41.2921, -5.559) ccw
  arc A185 (42.0628, 17.2696) -> (41.1941, 19.2502) centre (0, 0) ccw
  arc A186 (38.0004, 13.748) -> (42.0628, 17.2696) centre (23.8765, 34.1446) ccw
  arc A187 (38.4318, 12.4912) -> (38.0004, 13.748) centre (0, 0) ccw
  arc A188 (43.8007, 12.2073) -> (38.4318, 12.4912) centre (39.8139, -12.2796) ccw
  arc A189 (44.3316, 10.1108) -> (43.8007, 12.2073) centre (0, 0) ccw
  arc A190 (39.745, 7.3058) -> (44.3316, 10.1108) centre (29.1709, 29.7489) ccw
  arc A191 (39.9637, 5.9952) -> (39.745, 7.3058) centre (0, 0) ccw
  arc A192 (45.2126, 4.8315) -> (39.9637, 5.9952) centre (37.2498, -18.6653) ccw
  arc A193 (45.3912, 2.6762) -> (45.2126, 4.8315) centre (0, 0) ccw
  arc A194 (40.4054, 0.6644) -> (45.3912, 2.6762) centre (33.6695, 24.5418) ccw
  arc A195 (40.4054, -0.6644) -> (40.4054, 0.6644) centre (0, 0) ccw
  arc A196 (45.3912, -2.6762) -> (40.4054, -0.6644) centre (33.6695, -24.5418) ccw
  arc A197 (45.2126, -4.8315) -> (45.3912, -2.6762) centre (0, 0) ccw
  arc A198 (39.9637, -5.9952) -> (45.2126, -4.8315) centre (37.2498, 18.6653) ccw
  arc A199 (39.745, -7.3058) -> (39.9637, -5.9952) centre (0, 0) ccw
  arc A200 (44.3316, -10.1108) -> (39.745, -7.3058) centre (29.1709, -29.7489) ccw
  arc A201 (43.8007, -12.2073) -> (44.3316, -10.1108) centre (0, 0) ccw
  arc A202 (38.4318, -12.4912) -> (43.8007, -12.2073) centre (39.8139, 12.2796) ccw
  arc A203 (38.0004, -13.748) -> (38.4318, -12.4912) centre (0, 0) ccw
  arc A204 (42.0628, -17.2696) -> (38.0004, -13.748) centre (23.8765, -34.1446) ccw
  arc A205 (41.1941, -19.2502) -> (42.0628, -17.2696) centre (0, 0) ccw
  arc A206 (35.8517, -18.6465) -> (41.1941, -19.2502) centre (41.2921, 5.559) ccw
  arc A207 (35.2193, -19.8151) -> (35.8517, -18.6465) centre (0, 0) ccw
  arc A208 (38.6466, -23.9574) -> (35.2193, -19.8151) centre (17.9308, -37.6088) ccw
  arc A209 (37.4637, -25.768) -> (38.6466, -23.9574) centre (0, 0) ccw
  arc A210 (32.2936, -24.2932) -> (37.4637, -25.768) centre (41.6439, -1.3133) ccw
  arc A211 (31.4775, -25.3418) -> (32.2936, -24.2932) centre (0, 0) ccw
  arc A212 (34.1763, -29.9917) -> (31.4775, -25.3418) centre (11.4961, -40.0472) ccw
  arc A213 (32.7115, -31.5829) -> (34.1763, -29.9917) centre (0, 0) ccw
  arc A214 (27.8546, -29.2772) -> (32.7115, -31.5829) centre (40.8598, -8.1497) ccw
  arc A215 (26.877, -30.1772) -> (27.8546, -29.2772) centre (0, 0) ccw
  arc A216 (28.7737, -35.2079) -> (26.877, -30.1772) centre (4.7477, -41.3932) ccw
  arc A217 (27.067, -36.5363) -> (28.7737, -35.2079) centre (0, 0) ccw
  arc A218 (22.6558, -33.4627) -> (27.067, -36.5363) centre (38.9611, -14.7639) ccw
  arc A219 (21.5435, -34.1894) -> (22.6558, -33.4627) centre (0, 0) ccw
  arc A220 (22.5862, -39.4637) -> (21.5435, -34.1894) centre (-2.1301, -41.6101) ccw
  arc A221 (20.6842, -40.493) -> (22.5862, -39.4637) centre (0, 0) ccw
  arc A222 (16.8391, -36.7353) -> (20.6842, -40.493) centre (35.9996, -20.9753) ccw
  arc A223 (15.6222, -37.269) -> (16.8391, -36.7353) centre (0, 0) ccw
  arc A224 (15.7827, -42.643) -> (15.6222, -37.269) centre (-8.9499, -40.692) ccw
  arc A225 (13.7371, -43.3453) -> (15.7827, -42.643) centre (0, 0) ccw
  arc A226 (10.563, -39.0059) -> (13.7371, -43.3453) centre (32.0562, -26.6146) ccw
  arc A227 (9.2749, -39.3321) -> (10.563, -39.0059) centre (0, 0) ccw
  arc A228 (8.5486, -44.6592) -> (9.2749, -39.3321) centre (-15.5255, -38.6639) ccw
  arc A229 (6.4154, -45.0151) -> (8.5486, -44.6592) centre (0, 0) ccw
  arc A230 (3.9987, -40.2125) -> (6.4154, -45.0151) centre (27.2384, -31.5279) ccw
  arc A231 (2.6745, -40.3222) -> (3.9987, -40.2125) centre (0, 0) ccw
  arc A232 (1.0814, -45.4571) -> (2.6745, -40.3222) centre (-21.6776, -35.5812) ccw
  arc A233 (-1.0814, -45.4571) -> (1.0814, -45.4571) centre (0, 0) ccw
  arc A234 (-2.6745, -40.3222) -> (-1.0814, -45.4571) centre (21.6776, -35.5812) ccw
  arc A235 (-3.9987, -40.2125) -> (-2.6745, -40.3222) centre (0, 0) ccw
  arc A236 (-6.4154, -45.0151) -> (-3.9987, -40.2125) centre (-27.2384, -31.5279) ccw
  arc A237 (-8.5486, -44.6592) -> (-6.4154, -45.0151) centre (0, 0) ccw
  arc A238 (-9.2749, -39.3321) -> (-8.5486, -44.6592) centre (15.5255, -38.6639) ccw
  arc A239 (-10.563, -39.0059) -> (-9.2749, -39.3321) centre (0, 0) ccw
  arc A240 (-13.7371, -43.3453) -> (-10.563, -39.0059) centre (-32.0562, -26.6146) ccw
  arc A241 (-15.7827, -42.643) -> (-13.7371, -43.3453) centre (0, 0) ccw
  arc A242 (-15.6222, -37.269) -> (-15.7827, -42.643) centre (8.9499, -40.692) ccw
  arc A243 (-16.8391, -36.7353) -> (-15.6222, -37.269) centre (0, 0) ccw
  arc A244 (-20.6842, -40.493) -> (-16.8391, -36.7353) centre (-35.9996, -20.9753) ccw
  arc A245 (-22.5862, -39.4637) -> (-20.6842, -40.493) centre (0, 0) ccw
  arc A246 (-21.5435, -34.1894) -> (-22.5862, -39.4637) centre (2.1301, -41.6101) ccw
  arc A247 (-22.6558, -33.4627) -> (-21.5435, -34.1894) centre (0, 0) ccw
  arc A248 (-27.067, -36.5363) -> (-22.6558, -33.4627) centre (-38.9611, -14.7639) ccw
  arc A249 (-28.7737, -35.2079) -> (-27.067, -36.5363) centre (0, 0) ccw
  arc A250 (-26.877, -30.1772) -> (-28.7737, -35.2079) centre (-4.7477, -41.3932) ccw
  arc A251 (-27.8546, -29.2772) -> (-26.877, -30.1772) centre (0, 0) ccw
  arc A252 (-32.7115, -31.5829) -> (-27.8546, -29.2772) centre (-40.8598, -8.1497) ccw
  arc A253 (-34.1763, -29.9917) -> (-32.7115, -31.5829) centre (0, 0) ccw
  arc A254 (-31.4775, -25.3418) -> (-34.1763, -29.9917) centre (-11.4961, -40.0472) ccw
  arc A255 (-32.2936, -24.2932) -> (-31.4775, -25.3418) centre (0, 0) ccw
  arc A256 (-37.4637, -25.768) -> (-32.2936, -24.2932) centre (-41.6439, -1.3133) ccw
  arc A257 (-38.6466, -23.9574) -> (-37.4637, -25.768) centre (0, 0) ccw
  arc A258 (-35.2193, -19.8151) -> (-38.6466, -23.9574) centre (-17.9308, -37.6088) ccw
  arc A259 (-35.8517, -18.6465) -> (-35.2193, -19.8151) centre (0, 0) ccw
  arc A260 (-41.1941, -19.2502) -> (-35.8517, -18.6465) centre (-41.2921, 5.559) ccw
  arc A261 (-42.0628, -17.2696) -> (-41.1941, -19.2502) centre (0, 0) ccw
  arc A262 (-38.0004, -13.748) -> (-42.0628, -17.2696) centre (-23.8765, -34.1446) ccw
  arc A263 (-38.4318, -12.4912) -> (-38.0004, -13.748) centre (0, 0) ccw
  arc A264 (-43.8007, -12.2073) -> (-38.4318, -12.4912) centre (-39.8139, 12.2796) ccw
  arc A265 (-44.3316, -10.1108) -> (-43.8007, -12.2073) centre (0, 0) ccw
  arc A266 (-39.745, -7.3058) -> (-44.3316, -10.1108) centre (-29.1709, -29.7489) ccw
  arc A267 (-39.9637, -5.9952) -> (-39.745, -7.3058) centre (0, 0) ccw
  arc A268 (-45.2126, -4.8315) -> (-39.9637, -5.9952) centre (-37.2498, 18.6653) ccw
  arc A269 (-45.3912, -2.6762) -> (-45.2126, -4.8315) centre (0, 0) ccw
  arc A270 (-40.4054, -0.6644) -> (-45.3912, -2.6762) centre (-33.6695, -24.5418) ccw
  arc A271 (-40.4054, 0.6644) -> (-40.4054, -0.6644) centre (0, 0) ccw
  arc A272 (-45.3912, 2.6762) -> (-40.4054, 0.6644) centre (-33.6695, 24.5418) ccw
  arc A273 (-45.2126, 4.8315) -> (-45.3912, 2.6762) centre (0, 0) ccw
  arc A274 (-39.9637, 5.9952) -> (-45.2126, 4.8315) centre (-37.2498, -18.6653) ccw
  arc A275 (-39.745, 7.3058) -> (-39.9637, 5.9952) centre (0, 0) ccw
  arc A276 (-44.3316, 10.1108) -> (-39.745, 7.3058) centre (-29.1709, 29.7489) ccw
  arc A277 (-43.8007, 12.2073) -> (-44.3316, 10.1108) centre (0, 0) ccw
  arc A278 (-38.4318, 12.4912) -> (-43.8007, 12.2073) centre (-39.8139, -12.2796) ccw
  arc A279 (-38.0004, 13.748) -> (-38.4318, 12.4912) centre (0, 0) ccw
  arc A280 (-42.0628, 17.2696) -> (-38.0004, 13.748) centre (-23.8765, 34.1446) ccw
  arc A281 (-41.1941, 19.2502) -> (-42.0628, 17.2696) centre (0, 0) ccw
  arc A282 (-35.8517, 18.6465) -> (-41.1941, 19.2502) centre (-41.2921, -5.559) ccw
  arc A283 (-35.2193, 19.8151) -> (-35.8517, 18.6465) centre (0, 0) ccw
  arc A284 (-38.6466, 23.9574) -> (-35.2193, 19.8151) centre (-17.9308, 37.6088) ccw
  arc A285 (-37.4637, 25.768) -> (-38.6466, 23.9574) centre (0, 0) ccw
  arc A286 (-32.2936, 24.2932) -> (-37.4637, 25.768) centre (-41.6439, 1.3133) ccw
  arc A287 (-31.4775, 25.3418) -> (-32.2936, 24.2932) centre (0, 0) ccw
  arc A288 (-34.1763, 29.9917) -> (-31.4775, 25.3418) centre (-11.4961, 40.0472) ccw
  arc A289 (-32.7115, 31.5829) -> (-34.1763, 29.9917) centre (0, 0) ccw
  arc A290 (-27.8546, 29.2772) -> (-32.7115, 31.5829) centre (-40.8598, 8.1497) ccw
  arc A291 (-26.877, 30.1772) -> (-27.8546, 29.2772) centre (0, 0) ccw
  arc A292 (-28.7737, 35.2079) -> (-26.877, 30.1772) centre (-4.7477, 41.3932) ccw
  arc A293 (-27.067, 36.5363) -> (-28.7737, 35.2079) centre (0, 0) ccw
  arc A294 (-22.6558, 33.4627) -> (-27.067, 36.5363) centre (-38.9611, 14.7639) ccw
  arc A295 (-21.5435, 34.1894) -> (-22.6558, 33.4627) centre (0, 0) ccw
  arc A296 (-22.5862, 39.4637) -> (-21.5435, 34.1894) centre (2.1301, 41.6101) ccw
  arc A297 (-20.6842, 40.493) -> (-22.5862, 39.4637) centre (0, 0) ccw
  arc A298 (-16.8391, 36.7353) -> (-20.6842, 40.493) centre (-35.9996, 20.9753) ccw
  arc A299 (-15.6222, 37.269) -> (-16.8391, 36.7353) centre (0, 0) ccw
  arc A300 (-15.7827, 42.643) -> (-15.6222, 37.269) centre (8.9499, 40.692) ccw
  arc A301 (-13.7371, 43.3453) -> (-15.7827, 42.643) centre (0, 0) ccw
  arc A302 (-10.563, 39.0059) -> (-13.7371, 43.3453) centre (-32.0562, 26.6146) ccw
  arc A303 (-9.2749, 39.3321) -> (-10.563, 39.0059) centre (0, 0) ccw
  arc A304 (-8.5486, 44.6592) -> (-9.2749, 39.3321) centre (15.5255, 38.6639) ccw
  arc A305 (-6.4154, 45.0151) -> (-8.5486, 44.6592) centre (0, 0) ccw
  arc A306 (-3.9987, 40.2125) -> (-6.4154, 45.0151) centre (-27.2384, 31.5279) ccw
  arc A307 (-2.6745, 40.3222) -> (-3.9987, 40.2125) centre (0, 0) ccw
  arc A308 (-1.0814, 45.4571) -> (-2.6745, 40.3222) centre (21.6776, 35.5812) ccw
  circle A309 centre (-12, 12) radius 2.72
  circle A310 centre (0, 0) radius 5.22
  circle A311 centre (-12, -12) radius 2.72
  circle A312 centre (12, 12) radius 2.72
  circle A313 centre (12, -12) radius 2.72
  constraints: 308 other